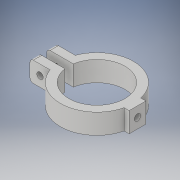
# Autodesk Inventor part: CameraClamp
Saved by Autodesk Inventor 2019 (Build 230136000, 136)
## iProperties
Created: 2019-07-15
Part Number: CameraClamp
Material: Generic
Document SubType Name: Modeling
Designer: aorfi
Density: 1 g/cm^3
Appearance: Default
Author: aorfi
Autodesk Inventor part; units mm, degrees
ref_plane "XZ Plane" through (0, 0, 0) normal (0, 1, 0) x (-1, 0, 0)
ref_plane "XY Plane" through (0, 0, 0) normal (0, 0, 1) x (1, 0, 0)
sketch "Sketch1" plane through (0, 0, 0) normal (0, 1, 0) x (-1, 0, 0)
  arc A0 (16.5624, 2.5) -> (16.5624, -2.5) centre (0, 0) ccw
  arc A1 (20.416, 7.5) -> (20.416, -7.5) centre (0, 0) ccw
  line L0 (32.416, 7.5) -> (20.416, 7.5)
  line L1 (16.5624, 2.5) -> (32.416, 2.5)
  line L2 (32.416, 2.5) -> (32.416, 7.5)
  line L3 (32.416, -2.5) -> (16.5624, -2.5)
  line L4 (20.416, -7.5) -> (32.416, -7.5)
  line L5 (32.416, -7.5) -> (32.416, -2.5)
  line L6 (26.416, 5) -> (26.416, -5) construction
  line L7 (-21.1675, -5) -> (-24.1675, -5)
  line L8 (-24.1675, -5) -> (-24.1675, 5)
  line L9 (-24.1675, 5) -> (-21.1675, 5)
  line L10 (-21.1675, 5) -> (-21.1675, -5)
  point P0 (32.416, 5)
  point P1 (32.416, -5)
  point P2 (26.416, 0)
  point P3 (26.416, -7.5)
  point P4 (-16.75, 0)
  point P5 (-24.1675, 0)
  dimension "d0" = 33.5
  dimension "d1" = 5
  dimension "d4" = 5
  dimension "d5" = 5
  dimension "d6" = 10
  dimension "d7" = 12
  dimension "d35" = 10
  dimension "d36" = 3
  constraints: 22 end point, 6 point on circle, 5 midpoint, 4 horizontal alignment, 4 parallel, 3 horizontal, 3 vertical, 2 centre point, 1 coincident, 1 perpendicular, 1 point on line, 1 vertical alignment
  measures "d0" diameter of A0
  measures "d1" radial gap between concentric circles of A0 A1
  measures "d4" distance of L1.end L0.start
  measures "d5" distance of L4.end L3.start
  measures "d6" distance of L6.start L6.end
  measures "d7" distance of L4.start L4.end
  measures "d35" distance of L7.end L8.end
  measures "d36" distance of L8.end L9.end
extrude "Extrusion1" add sketch "Sketch1" along normal mid plane 12
sketch "Sketch2" plane through (-32.416, 6, 7.5) normal (0, 0, 1) x (1, 0, 0)
  line L0 (0, 0) -> (0, -12) projected
  line L1 (0, 0) -> (12, 0) projected
  point P0 (32.416, -6)
  point P1 (6, -6)
  point P2 (0, -6)
  point P3 (6, 0)
  constraints: 2 midpoint, 1 horizontal alignment, 1 vertical alignment
hole "Hole1" at (-26.416, 0, 7.5) direction (0, 0, -1) diameter 3.797 depth 5 clearance for "Flat Head Machine Screw (82)" size "#6" standard "Ansi Unified Screw Threads"
sketch "Sketch3" plane through (-20.416, 6, -7.5) normal (0, 0, -1) x (-1, 0, 0)
  line L0 (8.3161, -1.9884) -> (10.6322, -6)
  line L1 (10.6322, -6) -> (8.3161, -10.0116)
  line L2 (8.3161, -10.0116) -> (3.6839, -10.0116)
  line L3 (3.6839, -10.0116) -> (1.3678, -6)
  line L4 (1.3678, -6) -> (3.6839, -1.9884)
  line L5 (3.6839, -1.9884) -> (8.3161, -1.9884)
  circle A0 centre (6, -6) radius 1.8985 projected
  point P0 (-20.416, -6)
  dimension "d17" = 8.0232
  constraints: 12 end point, 1 coincident, 1 horizontal, 13 other
  measures "d17" distance between parallel lines of L5 L2
extrude "Extrusion2" [suppressed]
fillet "Fillet1" radius 2 4 edges at (-32.416, -6, -5) (-32.416, 6, -5) (-32.416, 6, 5) (-32.416, -6, 5)
ref_plane "Work Plane3" through (19.75, 0, 0) normal (1, 0, 0) x (0, 1, 0)
sketch "Sketch5" plane through (19.75, 0, 0) normal (1, 0, 0) x (0, 1, 0)
  circle A0 centre (0, 0) radius 3.25
  dimension "d25" = 6.5
  constraints: 1 centre point, 1 coincident
  measures "d25" diameter of A0
extrude "Extrusion4" cut sketch "Sketch5" against normal up to next
hole "Hole2" at (19.75, 0, 0) direction (1, 0, 0) diameter 3.797 end through all clearance for "Flat Head Machine Screw (82)" size "#6" standard "Ansi Unified Screw Threads"
sketch "Sketch6" plane through (-20.416, -6, -7.5) normal (0, 0, -1) x (-1, 0, 0)
  line L0 (10, 0) -> (-3.8536, 0) projected
  point P0 (-20.416, 6)
  point P1 (6, 6)
hole "Hole3" at (-26.416, 0, -7.5) direction (0, 0, 1) diameter 2.642 depth 5 thread size "6-32 UNC" class "2B" standard "ANSI Unified Screw Threads"
equation "\"d5\" = d4"
body "Solid1"
